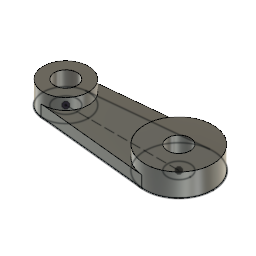
link (Autodesk Fusion 360 design; units mm, degrees)
Autodesk Fusion 360 part; units mm, degrees
note: some values were not read from the file. Set by a fixed rule: the direction of a hole.
sketch "Sketch1" plane through (0, 0, 0) normal (0, 0, 1) x (1, 0, 0)
  line L0 (0, 0) -> (100, 0) construction
  line L1 (100, 0) -> (0, 0) construction
  circle A0 centre (0, 0) radius 20
  circle A1 centre (100, 0) radius 30
  line L2 (-2, 19.8997) -> (97, 29.8496)
  line L3 (-2, -19.8997) -> (97, -29.8496)
  circle A2 centre (0, 0) radius 10
  circle A3 centre (100, 0) radius 10
  dimension "d1" = 100
  dimension "d2" = 40
  dimension "d3" = 60
  dimension "d4" = 20
  dimension "d5" = 20
  constraint coincident L0.start L1.end
  constraint horizontal L0
  constraint coincident L0.end L1.start
  constraint coincident A0 L2.start
  constraint coincident A1 L2.end
  constraint coincident A0 L3.start
  constraint coincident A1 L3.end
  constraint tangent A0 L2
  constraint tangent A1 L3
  constraint tangent A0 L3
  constraint tangent A1 L2
  constraint concentric A1 A3
  measures "d1" distance of L0.start L0.end
  measures "d2" diameter of A0
  measures "d3" diameter of A1
  measures "d4" diameter of A2
  measures "d5" diameter of A3
extrude "Extrude1" add sketch "Sketch1" along normal blind 20 contours A0 | A1 | A2 | A3 makes body 1 at (19.9006, -1.9914, 6.6667) makes body 2 at (129.8509, -2.987, 6.6667)
extrude "Extrude2" add sketch "Sketch1" along normal blind 10 contours A0 A1 L2 L3 bodies 1 2
hole "Hole1" at (100, 0, 0) direction (0, 0, 1) diameter 20 depth 40 tip angle 180 bodies 1
hole "Hole2" at (0, 0, 0) direction (0, 0, 1) diameter 20 end through all bodies 1
